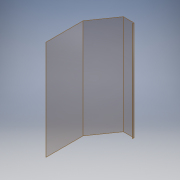
# Autodesk Inventor part: polycarbonate cover
Saved by Autodesk Inventor 2018 (Build 220112000, 112)
## iProperties
Created: 2018-04-10
Part Number: polycarbonate cover
Material: Polycarbonate, Smoke
Document SubType Name: Modeling
Designer: P446509
Density: 1.2 g/cm^3
Appearance: Polycarbonate - Smoked
Author: P446509
Autodesk Inventor part; units mm, degrees
ref_plane "YZ Plane" through (0, 0, 0) normal (1, 0, 0) x (0, 1, 0)
ref_plane "XZ Plane" through (0, 0, 0) normal (0, 1, 0) x (-1, 0, 0)
ref_plane "XY Plane" through (0, 0, 0) normal (0, 0, 1) x (1, 0, 0)
sketch "Sketch1" plane through (0, 0, 0) normal (0, 0, 1) x (1, 0, 0)
  line L0 (0, -20) -> (0, 0)
  line L1 (0, 0) -> (-130, 0)
  line L2 (-130, 0) -> (-330.7518, -286.7032)
  line L3 (-330.7518, -286.7032) -> (-330.7518, -735.1242)
  line L4 (-326.7518, -735.1242) -> (-326.7518, -287.9644)
  line L5 (-326.7518, -287.9644) -> (-127.9177, -4)
  line L6 (-127.9177, -4) -> (-4, -4)
  line L7 (-4, -4) -> (-4, -20)
  line L8 (-4, -20) -> (0, -20)
  line L9 (-330.7518, -735.1242) -> (-326.7518, -735.1242)
  dimension "d0" = 20
  dimension "d1" = 130
  dimension "d2" = 125
  dimension "d3" = 350
  dimension "d4" = 448.421
  dimension "d5" = 4
  constraints: 20 end point, 3 parallel, 2 perpendicular, 1 horizontal, 1 vertical, 3 other
  measures "d0" distance of L0.start L0.end
  measures "d1" distance of L0.end L1.end
  measures "d2" angle of L1 L2
  measures "d3" distance of L1.end L2.end
  measures "d4" distance of L2.end L3.end
  measures "d5" distance between parallel lines of L2 L5
extrude "Extrusion1" add sketch "Sketch1" along normal blind 1200
body "Solid1"
